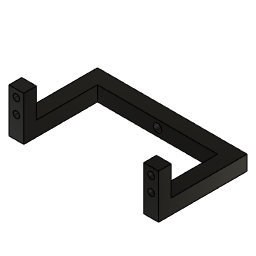
eye_blocker (Autodesk Fusion 360 archive; units mm, degrees)
design "blocker"
Autodesk Fusion 360 part; units mm, degrees
sketch "Sketch1" plane through (0, 0, 0) normal (0, 0, 1) x (1, 0, 0)
  line L0 (0, 0) -> (7, 0)
  line L1 (7, 0) -> (7, 35)
  line L2 (7, 35) -> (64, 35)
  line L3 (64, 35) -> (64, 0)
  line L4 (64, 0) -> (71, 0)
  line L5 (71, 0) -> (71, 42)
  line L6 (71, 42) -> (0, 42)
  line L7 (0, 42) -> (0, 0)
  dimension "d1" = 7
  dimension "d2" = 35
  dimension "d3" = 57
  dimension "d9" = 7
  constraint coincident L0.start L7.end
  constraint horizontal L0
  constraint perpendicular L0 L1
  constraint perpendicular L1 L2
  constraint perpendicular L2 L3
  constraint perpendicular L3 L4
  constraint perpendicular L4 L5
  constraint perpendicular L5 L6
  constraint perpendicular L4 L7
  constraint equal L0 L4
  measures "d1" distance of L0.start L0.end
  measures "d2" distance of L0.end L1.end
  measures "d3" distance of L1.end L2.end
  measures "d9" distance of L2 L6
extrude "Extrude1" add sketch "Sketch1" along normal blind 7
sketch "Sketch2" plane through (0, 0, 7) normal (0, 0, 1) x (-1, 0, 0)
  line L0 (0, -42) -> (0, 0)
  line L1 (0, 0) -> (-7, 0)
  line L2 (-7, 0) -> (-7, -35)
  line L3 (-7, -35) -> (-64, -35)
  line L4 (-64, -35) -> (-64, 0)
  line L5 (-64, 0) -> (-71, 0)
  line L6 (-71, 0) -> (-71, -42)
  line L7 (-71, -42) -> (0, -42)
  line L8 (0, -4) -> (-7, -4)
  line L9 (-64, -4) -> (-71, -4)
  dimension "d10" = 4
  constraint coincident L0 L8.start
  constraint coincident L2 L8.end
  constraint perpendicular L2 L8
  constraint coincident L4 L9.start
  constraint coincident L6 L9.end
  constraint perpendicular L6 L9
  measures "d10" distance of L1 L8
extrude "Extrude2" add sketch "Sketch2" along normal blind 7 contours L0 L1 L2 L8 | L4 L5 L6 L9
extrude "Extrude4" add 1 faces at (4.6667, 2.6667, 14) along direction (0, 0, 1) blind 7
extrude "Extrude5" add 1 faces at (66.3333, 2.6667, 14) along direction (0, 0, 1) blind 7
sketch "Sketch5" plane through (0, 42, 0) normal (0, 1, 0) x (-1, 0, 0)
  line L0 (-71, 0) -> (0, 0)
  line L1 (0, 0) -> (0, 7)
  line L2 (0, 7) -> (-71, 7)
  line L3 (-71, 7) -> (-71, 0)
  line L4 (-71, 7) -> (0, 0)
  line L5 (0, 7) -> (-71, 0)
  circle A0 centre (-35.5, 3.5) radius 2
  dimension "d25" = 4
  constraint coincident L2.end L3.start
  constraint coincident L0.end L1.start
  constraint coincident L1.end L2.start
  constraint coincident L0.start L3.end
  constraint midpoint L4 A0.centre
  measures "d25" diameter of A0
extrude "Extrude7" cut sketch "Sketch5" against normal blind 100 contours L4 L5 A0 | L4 L5 A0 | L4 L5 A0 | L4 L5 A0
sketch "Sketch6" plane through (0, 0, 0) normal (0, -1, 0) x (1, 0, 0)
  line L0 (0, 0) -> (7, 0)
  line L1 (7, 0) -> (7, 21)
  line L2 (7, 21) -> (0, 21)
  line L3 (0, 21) -> (0, 0)
  line L4 (3.5, 21) -> (3.5, 17.5)
  circle A0 centre (3.5, 17.5) radius 1.55
  line L5 (3.5, 17.5) -> (3.5, 10.5)
  circle A1 centre (3.5, 10.5) radius 1.55
  dimension "d28" = 3.5
  dimension "d29" = 3.1
  dimension "d30" = 7
  constraint midpoint L2 L4.start
  constraint perpendicular L2 L4
  constraint coincident L4.end A0.centre
  constraint parallel L4 L5
  constraint coincident L5.end A1.centre
  constraint equal A0 A1
  measures "d28" distance of L4.start L4.end
  measures "d29" diameter of A0
  measures "d30" distance of L4.end L5.end
sketch "Sketch7" plane through (0, 0, 0) normal (0, -1, 0) x (1, 0, 0)
  line L0 (64, 0) -> (71, 0)
  line L1 (71, 0) -> (71, 21)
  line L2 (71, 21) -> (64, 21)
  line L3 (64, 21) -> (64, 0)
  line L4 (67.5, 21) -> (67.5, 17.5)
  line L5 (67.5, 17.5) -> (67.5, 10.5)
  circle A0 centre (67.5, 17.5) radius 1.55
  circle A1 centre (67.5, 10.5) radius 1.55
  dimension "d31" = 3.5
  dimension "d32" = 7
  dimension "d33" = 3.1
  constraint midpoint L2 L4.start
  constraint perpendicular L2 L4
  constraint parallel L4 L5
  constraint coincident L4.end L5.start
  constraint coincident L5.end A1.centre
  constraint equal A0 A1
  measures "d31" distance of L4.start L4.end
  measures "d32" distance of L4.end L5.end
  measures "d33" diameter of A0
extrude "Extrude8" cut sketch "Sketch6" sketch "Sketch7" against normal blind 100 contours L4 A0 L5 | L4 A0 L5 | A1 of sketch 2 contours L4 L5 A0 | L4 L5 A0 | A1
extrude "Extrude9" add 2 faces at (6.327, 4, 15.0144) (64.673, 4, 15.0144) along direction (0, 1, 0) blind 2
